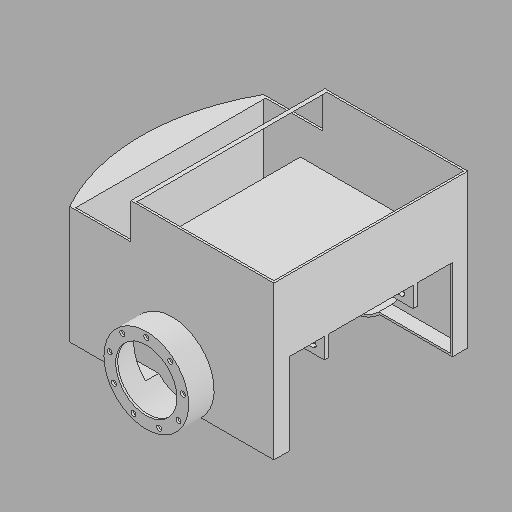
# Autodesk Inventor part: BODY
Saved by Autodesk Inventor 2025.2 (Build 292293000, 293)
## iProperties
Created: 2026-06-07
Part Number: BODY
Material: Generic
Document SubType Name: Modeling
Designer: Ben
Density: 1 g/cm^3
Appearance: Default
Mass: 225.699 g
Surface Area: 2299.79 cm^2
Volume: 225.699 cm^3
Author: Ben
Autodesk Inventor part; units mm, degrees
ref_plane "YZ Plane" through (0, 0, 0) normal (1, 0, 0) x (0, 1, 0)
ref_plane "XZ Plane" through (0, 0, 0) normal (0, 1, 0) x (-1, 0, 0)
ref_plane "XY Plane" through (0, 0, 0) normal (0, 0, 1) x (1, 0, 0)
sketch "Sketch1" plane through (0, 0, 0) normal (0, 0, 1) x (1, 0, 0)
  line L0 (-100, 75) -> (100, 75)
  line L1 (100, 75) -> (100, -75)
  line L2 (100, -75) -> (-100, -75)
  line L3 (-100, -75) -> (-100, 75)
  line L4 (-100, 75) -> (100, -75) construction
  line L5 (100, 75) -> (-100, -75) construction
  line L6 (-40, 75) -> (-100, 40)
  point P0 (0, 0)
  point P1 (-100, 0)
  dimension "d0" = 200
  dimension "d1" = 150
  dimension "d3" = 35
  dimension "d4" = 60
  constraints: 14 end point, 3 midpoint, 2 parallel, 2 point on line, 1 horizontal, 1 perpendicular
  measures "d0" distance of L0.start L0.end
  measures "d1" distance of L2.end L0.start
  measures "d3" distance from line of L6.end L0
  measures "d4" distance of L0.start L6.start
extrude "Extrusion1" add sketch "Sketch1" along normal mid plane 190 contours L0 L1 L2 L3 L6
sketch "Sketch4" plane through (0, 0, 95) normal (0, 0, 1) x (1, 0, 0)
  circle A0 centre (0, -45) radius 41.5
  point P0 (0, 0)
  dimension "d30" = 83
  dimension "d31" = 45
  constraints: 1 centre point, 1 vertical alignment
  measures "d30" diameter of A0
  measures "d31" distance of point (0, 0) A0.centre
extrude "Extrusion2" add sketch "Sketch4" along normal blind 25 and the other way blind 15
mirror "Mirror2" about plane through (0, 0, 0) normal (0, 0, 1) of "Extrusion2"
shell "Shell8" thickness 2 removed faces 3 at (6.6667, 75, 31.6667) at (-7.1699, -76.8302, 80) at (-7.1699, -76.8302, -80)
sketch "Sketch10" plane through (0, -45, 120) normal (0, 0, 1) x (1, 0, 0)
  circle A0 centre (0, 0) radius 30
  circle A1 centre (0, 0) radius 41.5 projected
  circle A2 centre (0, 36.5) radius 2.5
  circle A3 centre (-23.4617, 27.9606) radius 2.5
  circle A4 centre (-35.9455, 6.3382) radius 2.5
  circle A5 centre (-31.6099, -18.25) radius 2.5
  circle A6 centre (-12.4837, -34.2988) radius 2.5
  circle A7 centre (12.4837, -34.2988) radius 2.5
  circle A8 centre (31.6099, -18.25) radius 2.5
  circle A9 centre (35.9455, 6.3382) radius 2.5
  circle A10 centre (23.4617, 27.9606) radius 2.5
  point P0 (0, 45)
  dimension "d83" = 60
  dimension "d84" = 5
  dimension "d85" = 36.5
  dimension "d88" = 360
  constraints: 10 centre point, 1 concentric, 1 vertical alignment, 19 other
  measures "d83" diameter of A0
  measures "d84" diameter of A2
  measures "d85" distance of A0.centre A2.centre
extrude "Extrusion7" cut sketch "Sketch10" against normal up to surface (2 mm away) contours A0 | A2 | A3 | A4 | A5 | A6 | A7 | A8 | A9 | A10
mirror "Mirror3" about plane through (0, 0, 0) normal (0, 0, 1) of "Extrusion7"
sketch "Sketch11" plane through (100, -75, -95) normal (0, -1, 0) x (1, 0, 0)
  line L0 (0, 190) -> (0, 0) projected
  line L1 (0, 175) -> (-175, 175)
  line L2 (-175, 175) -> (-175, 15)
  line L3 (-175, 15) -> (0, 15)
  line L4 (0, 15) -> (0, 175)
  line L5 (-200, 0) -> (-200, 190) projected
  point P0 (-100, 95)
  point P1 (-71.3251, 175)
  point P2 (-128.6749, 15)
  point P3 (0, 15)
  dimension "d92" = 25
  constraints: 8 end point, 2 horizontal alignment, 2 parallel, 1 horizontal, 1 perpendicular, 1 point on line
  measures "d92" distance between parallel lines of L5 L2
extrude "Extrusion8" cut sketch "Sketch11" against normal blind 80
sketch "Sketch15" plane through (98, -73, 93) normal (-1, 0, 0) x (0, 0, 1)
  line L0 (2, -2) -> (2, 148) projected
  line L1 (-188, -2) -> (-188, 113) projected
  line L2 (2, 78) -> (-188, 78)
  line L3 (-188, 78) -> (-188, 80)
  line L4 (-188, 80) -> (2, 80)
  line L5 (2, 80) -> (2, 78)
  point P0 (-93, 73)
  point P1 (-173, 78)
  point P2 (-188, 78)
  dimension "d103" = 2
  constraints: 8 end point, 2 parallel, 2 point on line, 1 horizontal, 1 horizontal alignment, 1 perpendicular
  measures "d103" distance between parallel lines of L2 L4
extrude "Extrusion10" add sketch "Sketch15" along normal blind 160
sketch "Sketch16" plane through (100, 5, -95) normal (0, -1, 0) x (1, 0, 0)
  line L0 (0, 140.5) -> (-162, 140.5)
  line L1 (-162, 140.5) -> (-162, 136.5)
  line L2 (-162, 136.5) -> (0, 136.5)
  line L3 (0, 136.5) -> (0, 140.5)
  line L4 (0, 175) -> (0, 15) construction
  line L5 (0, 95) -> (-162, 95) construction
  line L6 (-162, 2) -> (-162, 188) construction
  line L7 (0, 49.5) -> (-162, 49.5)
  line L8 (-162, 49.5) -> (-162, 53.5)
  line L9 (-162, 53.5) -> (0, 53.5)
  line L10 (0, 53.5) -> (0, 49.5)
  point P0 (-100, 95)
  point P1 (-162, 95)
  dimension "d106" = 4
  dimension "d107" = 83
  constraints: 18 end point, 4 midpoint, 4 symmetric about line, 2 parallel, 2 vertical alignment, 1 horizontal, 1 perpendicular
  measures "d106" distance between parallel lines of L2 L0
  measures "d107" distance between parallel lines of L9 L2
extrude "Extrusion11" add sketch "Sketch16" along normal blind 20
sketch "Sketch17" plane through (-62, 5, 45.5) normal (0, 0, 1) x (1, 0, 0)
  line L0 (162, 0) -> (0, 0) projected
  line L1 (162, 0) -> (162, -20) projected
  line L2 (0, -20) -> (162, -20) projected
  line L3 (0, 0) -> (0, -20) projected
  line L4 (11, -12) -> (151, -12) construction
  line L5 (11, -15) -> (151, -15)
  line L6 (151, -9) -> (11, -9)
  arc A0 (11, -9) -> (11, -15) centre (11, -12) ccw
  arc A1 (151, -15) -> (151, -9) centre (151, -12) ccw
  point P0 (81, -12)
  point P1 (81, 0)
  dimension "d111" = 6
  dimension "d112" = 140
  dimension "d115" = 5
  constraints: 8 end point, 4 point on circle, 4 tangent, 2 centre point, 2 midpoint, 2 parallel, 1 vertical alignment
  measures "d111" distance between parallel lines of L5 L6
  measures "d112" distance of L6.start L6.end
  measures "d115" distance between parallel lines of L2 L5
extrude "Extrusion12" cut sketch "Sketch17" against normal up to surface (91 mm away) contours A0 L6 A1 L5
sketch "Sketch18" plane through (-100, -75, -95) normal (0, -1, 0) x (1, 0, 0)
  line L0 (0, 0) -> (0, 190) projected
  arc A0 (0, 190) -> (0, 0) centre (168, 95) ccw
  line L1 (0, 0) -> (0, 190)
  line L2 (0, 0) -> (0, 190) projected
  point P0 (100, 95)
  point P1 (0, 95)
  point P2 (-25, 95)
  point P3 (0, 95)
  dimension "d116" = 25
  constraints: 3 point on circle, 2 end point, 2 midpoint, 1 centre point, 1 collinear, 1 horizontal alignment
  measures "d116" distance of point (0, 95) point (-25, 95)
extrude "Extrusion13" add sketch "Sketch18" against normal blind 115
sketch "Sketch19" plane through (0, 0, 95) normal (0, 0, 1) x (1, 0, 0)
  line L0 (-40, 75) -> (-100, 40) projected
  line L1 (-100, 40) -> (-40, 40)
  line L2 (-40, 40) -> (-40, 75)
  line L3 (-40, 75) -> (-100, 40)
  line L4 (-98, 38.8513) -> (-36.0307, 75) projected
  point P0 (0, 0)
  constraints: 6 end point, 1 horizontal, 1 parallel, 1 perpendicular
extrude "Extrusion14" cut sketch "Sketch19" against normal through all
body "Solid1"
